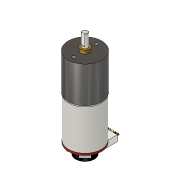
# Autodesk Inventor part: JGA25-371_12VDC_20RPM
Saved by Autodesk Inventor 2022 (Build 260153000, 153)
## iProperties
Created: 2022-08-15
Part Number: JGA25-371_12VDC_20RPM
Material: Generic
Document SubType Name: Modeling
Designer: Sebi
Density: 1 g/cm^3
Appearance: Default
Author: Sebi
Autodesk Inventor part; units mm, degrees
ref_plane "YZ Plane" through (0, 0, 0) normal (1, 0, 0) x (0, 1, 0)
ref_plane "XZ Plane" through (0, 0, 0) normal (0, 1, 0) x (-1, 0, 0)
ref_plane "XY Plane" through (0, 0, 0) normal (0, 0, 1) x (1, 0, 0)
sketch "Sketch1" plane through (0, 0, 0) normal (0, 1, 0) x (-1, 0, 0)
  circle A0 centre (0, 0) radius 12.2
  dimension "d0" = 24.4
  constraints: 1 centre point, 1 coincident
  measures "d0" diameter of A0
extrude "Extrusion1" add sketch "Sketch1" against normal blind 31
fillet "Fillet1" radius 1 1 edges at (12.2, 0, 0)
sketch "Sketch2" plane through (0, -31, 0) normal (0, -1, 0) x (1, 0, 0)
  circle A0 centre (0, 0) radius 12.2 projected
extrude "Extrusion2" add sketch "Sketch2" along normal blind 1.5 separate body
sketch "Sketch3" plane through (0, -32.5, 0) normal (0, -1, 0) x (1, 0, 0)
  circle A0 centre (0, 0) radius 7
  dimension "d6" = 14
  constraints: 1 centre point, 1 coincident
  measures "d6" diameter of A0
extrude "Extrusion3" add sketch "Sketch3" along normal blind 7.5 separate body
sketch "Sketch4" plane through (0, -32.5, 0) normal (0, -1, 0) x (1, 0, 0)
  circle A0 centre (0, 0) radius 6.75 construction
  line L0 (-7.4246, 2.8284) -> (-2.8284, 7.4246)
  line L1 (-2.8284, 7.4246) -> (-4.5962, 9.1924)
  line L2 (-4.5962, 9.1924) -> (-9.1924, 4.5962)
  line L3 (-9.1924, 4.5962) -> (-7.4246, 2.8284)
  line L4 (-7.4246, 2.8284) -> (-4.5962, 9.1924) construction
  line L5 (-2.8284, 7.4246) -> (-9.1924, 4.5962) construction
  line L6 (0, 0) -> (-6.0104, 6.0104) construction
  line L7 (0, 0) -> (-12.2, 0) construction
  circle A1 centre (0, 0) radius 12.2 construction
  point P0 (4.773, -4.773)
  dimension "d9" = 13.5
  dimension "d10" = 6.5
  dimension "d11" = 2.5
  dimension "d12" = 45
  dimension "d13" = 16.5
  constraints: 16 end point, 2 midpoint, 2 parallel, 2 perpendicular, 1 coincident, 1 horizontal, 1 horizontal alignment, 1 point on line, 4 other
  measures "d10" distance of L1.end L2.end
  measures "d11" distance of L0.end L1.end
  measures "d12" angle of L7 L6
  measures "d13" distance from line of point (4.773, -4.773) L2
extrude "Extrusion4" add sketch "Sketch4" along normal blind 3.5 separate body
pattern_circular "Circular Pattern1" count 2 over 90 about axis through (0, -32.5, 0) along (0, 1, 0) of "Extrusion4" bodies 4
sketch "Sketch5" plane through (0, -32.5, 0) normal (0, -1, 0) x (1, 0, 0)
  line L0 (-7.25, -17) -> (7.25, -17)
  line L1 (7.25, -17) -> (7.25, -8.5)
  line L2 (7.25, -8.5) -> (-7.25, -8.5)
  line L3 (-7.25, -8.5) -> (-7.25, -17)
  line L4 (-7.25, -17) -> (7.25, -8.5) construction
  line L5 (7.25, -17) -> (-7.25, -8.5) construction
  circle A0 centre (0, 0) radius 7 projected
  point P0 (0, -12.75)
  point P1 (0, -12.75)
  dimension "d19" = 17
  dimension "d20" = 8.5
  dimension "d21" = 14.5
  constraints: 12 end point, 3 midpoint, 2 parallel, 1 horizontal, 1 perpendicular, 1 vertical alignment
  measures "d19" distance from line of A0.centre L0
  measures "d20" distance of L2.end L0.start
  measures "d21" distance of L1.end L2.end
extrude "Extrusion5" add sketch "Sketch5" along normal blind 4.5 separate body contours L3 L2 L1 L0
sketch "Sketch6" plane through (7.25, -32.5, -17) normal (0, 0, -1) x (-1, 0, 0)
  line L0 (12.05, -2.25) -> (10.13, -2.25) construction
  line L1 (10.13, -2.25) -> (8.21, -2.25) construction
  line L2 (8.21, -2.25) -> (6.29, -2.25) construction
  line L3 (6.29, -2.25) -> (4.37, -2.25) construction
  line L4 (4.37, -2.25) -> (2.45, -2.25) construction
  circle A0 centre (12.05, -2.25) radius 0.7
  circle A1 centre (10.13, -2.25) radius 0.7
  circle A2 centre (8.21, -2.25) radius 0.7
  circle A3 centre (6.29, -2.25) radius 0.7
  circle A4 centre (4.37, -2.25) radius 0.7
  circle A5 centre (2.45, -2.25) radius 0.7
  line L5 (14.5, 0) -> (14.5, -4.5) projected
  line L6 (14.5, -4.5) -> (0, -4.5) projected
  point P0 (7.25, 32.5)
  point P1 (14.5, -2.25)
  point P2 (7.25, -2.25)
  point P3 (7.25, -4.5)
  dimension "d24" = 9.6
  dimension "d25" = 1.4
  constraints: 10 end point, 6 centre point, 6 coincident, 5 equal radius, 4 collinear, 4 point on line, 3 midpoint, 1 horizontal, 1 horizontal alignment, 1 vertical alignment
  measures "d24" distance of L4.end L0.start
  measures "d25" diameter of A0
extrude "Extrusion6" add sketch "Sketch6" along normal blind 3 separate body contours A0
extrude "Extrusion7" add sketch "Sketch6" along normal blind 3 separate body contours A1
extrude "Extrusion8" add sketch "Sketch6" along normal blind 3 separate body contours A2
extrude "Extrusion9" add sketch "Sketch6" along normal blind 3 separate body contours A3
extrude "Extrusion10" add sketch "Sketch6" along normal blind 3 separate body contours A4
extrude "Extrusion11" add sketch "Sketch6" along normal blind 3 separate body contours A5
sketch "Sketch7" plane through (0, 0, 0) normal (0, 1, 0) x (1, 0, 0)
  circle A0 centre (0, 0) radius 12.5
  dimension "d38" = 25
  constraints: 1 centre point, 1 coincident
  measures "d38" diameter of A0
extrude "Extrusion12" add sketch "Sketch7" along normal blind 27 separate body
sketch "Sketch8" plane through (0, 27, 0) normal (0, 1, 0) x (1, 0, 0)
  circle A0 centre (0, 0) radius 11.2 construction
  circle A1 centre (0, 0) radius 3.5
  dimension "d41" = 7
  constraints: 1 centre point, 1 coincident
  measures "d41" diameter of A1
extrude "Extrusion13" add sketch "Sketch8" along normal blind 2.5 separate body
sketch "Sketch9" plane through (0, 29.5, 0) normal (0, 1, 0) x (1, 0, 0)
  circle A0 centre (0, 0) radius 2
  dimension "d44" = 4
  constraints: 1 centre point, 1 coincident
  measures "d44" diameter of A0
extrude "Extrusion14" add sketch "Sketch9" along normal blind 9.5 separate body
chamfer "Chamfer1" distance 0.25 angle 45 1 edges at (-2, 39, 0)
sketch "Sketch10" plane through (0, 39, 0) normal (0, 1, 0) x (1, 0, 0)
  line L0 (-1.3229, -2) -> (1.3229, -2)
  line L1 (1.3229, -2) -> (1.3229, -1.5)
  line L2 (1.3229, -1.5) -> (-1.3229, -1.5)
  line L3 (-1.3229, -1.5) -> (-1.3229, -2)
  circle A0 centre (0, 0) radius 2 construction
  dimension "d50" = 1.5
  constraints: 8 end point, 2 parallel, 2 point on circle, 1 horizontal, 1 perpendicular, 1 tangent
  measures "d50" distance from line of point (0, 0) L2
extrude "Extrusion15" cut sketch "Sketch10" against normal blind 8 bodies 14
sketch "Sketch11" plane through (0, 27, 0) normal (0, 1, 0) x (1, 0, 0)
  circle A0 centre (0, 0) radius 12.5 construction
  line L0 (0, 8.5) -> (0, -8.5) construction
  line L1 (7.25, 8.5) -> (-7.25, 8.5) construction
  dimension "d53" = 17
  constraints: 3 coincident, 2 end point, 1 midpoint, 1 vertical
  measures "d53" distance of L0.start L0.end
hole "Hole1" at (0, 27, -8.5) at (0, 27, 8.5) direction (0, -1, 0) diameter 2.459 depth 8.8 tip angle 118 bodies 12 thread size "M3x0.5" class "6H" standard "ISO Metric profile"
body "Solid1"
body "Solid2"
body "Solid3"
body "Solid4"
body "Solid5"
body "Solid6"
body "Solid7"
body "Solid8"
body "Solid9"
body "Solid10"
body "Solid11"
body "Solid12"
body "Solid13"
body "Solid14"
